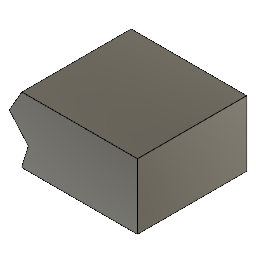
bear_moire (Autodesk Fusion 360 design; units mm, degrees)
Autodesk Fusion 360 part; units mm, degrees
sketch "Sketch1" plane through (0, 0, 0) normal (0, 1, 0) x (1, 0, 0)
  line L0 (0, 0) -> (-52.935, 0)
  line L1 (0, -30) -> (0, 0)
  line L2 (-52.935, 0) -> (-52.935, -0.4)
  line L3 (-52.9194, -30) -> (0, -30)
  line L4 (-52.935, -0.4) -> (-50, -10)
  line L5 (-50, -10) -> (-58.6929, -20)
  line L6 (-58.6929, -20) -> (-52.9194, -30)
  line L7 (-58.6929, -20) -> (0, -20) construction
  line L8 (-50, -10) -> (0, -10) construction
  line L9 (-29.3464, -20) -> (-29.3464, -30) construction
  line L10 (-29.3464, -20) -> (-29.3464, -10) construction
  line L11 (-29.3464, -10) -> (-29.3464, 0) construction
  dimension "d7" = 0.4
  dimension "d8" = 30
  dimension "d10" = 73
  dimension "d16" = 49
  dimension "d17" = 60
  dimension "d19" = 50
  constraint coincident L0.start L1.end
  constraint horizontal L0
  constraint perpendicular L0 L1
  constraint perpendicular L0 L2
  constraint perpendicular L1 L3
  constraint coincident L1 L7.end
  constraint perpendicular L1 L7
  constraint coincident L1 L8.end
  constraint perpendicular L1 L8
  constraint midpoint L7 L9.start
  constraint coincident L3 L9.end
  constraint perpendicular L3 L9
  constraint coincident L8 L10.end
  constraint perpendicular L8 L10
  constraint coincident L0 L11.end
  constraint perpendicular L0 L11
  constraint equal L10 L11
  constraint equal L9 L10
  measures "d7" distance of L2.end L0.end
  measures "d8" distance of L0 L3
  measures "d10" angle of L0 L4
  measures "d16" angle of L0 L5
  measures "d17" angle of L0 L6
  measures "d19" distance of L4.end L8.end
extrude "Extrude1" add sketch "Sketch1" along normal blind 50
equation "d7 = ( 0.2 * 2 ) * 1 mm"
